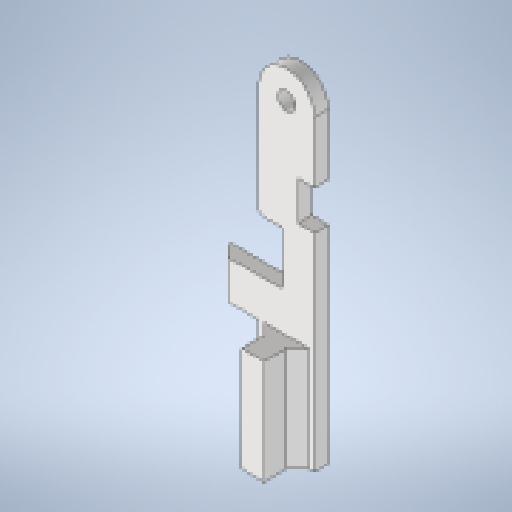
# Autodesk Inventor part: LatchLock
Saved by Autodesk Inventor 2025.1 (Build 291241000, 241)
## iProperties
Created: 2026-05-10
Part Number: LatchLock
Material: Generic
Document SubType Name: Modeling
Designer: User
Density: 1 g/cm^3
Appearance: Default
Author: User
Autodesk Inventor part; units mm, degrees
ref_plane "YZ Plane" through (0, 0, 0) normal (1, 0, 0) x (0, 1, 0)
ref_plane "XZ Plane" through (0, 0, 0) normal (0, 1, 0) x (-1, 0, 0)
ref_plane "XY Plane" through (0, 0, 0) normal (0, 0, 1) x (1, 0, 0)
sketch "Sketch1" plane through (0, 0, 0) normal (0, 0, 1) x (1, 0, 0)
  line L0 (8.404, 3) -> (8.404, -46.6888) projected
  line L1 (6.389, 0.2) -> (6.389, -55.1706) projected
  line L2 (7.404, -64.4706) -> (6.389, -64.4706) projected
  line L3 (6.389, -64.4706) -> (6.389, -78.3802) projected
  line L4 (-3.1786, -78.3802) -> (6.389, -78.3802) projected
  line L5 (-3.1786, -78.3802) -> (-3.1786, -81.1802) projected
  line L6 (8.404, -81.1802) -> (-3.1786, -81.1802) projected
  line L7 (8.404, -65.4706) -> (8.404, -81.1802) projected
  line L8 (8.604, -55.6706) -> (6.189, -55.6706)
  line L9 (6.189, -55.6706) -> (6.189, 0)
  line L10 (6.189, 0) -> (-3.3786, 0)
  line L11 (-3.3786, 0) -> (-3.3786, 3.2)
  line L12 (-3.3786, 3.2) -> (8.604, 3.2)
  line L13 (8.604, 3.2) -> (8.604, -55.6706)
  line L14 (8.604, -81.3802) -> (-3.3786, -81.3802)
  line L15 (-3.3786, -81.3802) -> (-3.3786, -78.1802)
  line L16 (-3.3786, -78.1802) -> (6.189, -78.1802)
  line L17 (6.189, -78.1802) -> (6.189, -64.2706)
  line L18 (6.189, -64.2706) -> (8.604, -64.2706)
  line L19 (8.604, -64.2706) -> (8.604, -81.3802)
  line L20 (13.604, -60.6706) -> (1.189, -60.6706)
  line L21 (1.189, -60.6706) -> (1.189, -5)
  line L22 (1.189, -5) -> (-8.3786, -5)
  line L23 (-8.3786, -5) -> (-8.3786, 8.2)
  line L24 (-8.3786, 8.2) -> (13.604, 8.2)
  line L25 (13.604, 8.2) -> (13.604, -60.6706)
  circle A0 centre (13.604, -26.2353) radius 5
  line L26 (18.604, -65.6706) -> (-3.811, -65.6706)
  line L27 (-3.811, -65.6706) -> (-3.811, -10)
  line L28 (-3.811, -10) -> (-13.3786, -10)
  line L29 (-13.3786, -10) -> (-13.3786, 13.2)
  line L30 (-13.3786, 13.2) -> (18.604, 13.2)
  line L31 (18.604, 13.2) -> (18.604, -65.6706)
  circle A1 centre (13.604, -26.2353) radius 1.6
  circle A2 centre (13.604, -26.2353) radius 30.3549
  circle A3 centre (13.604, -26.2353) radius 38.3626
  line L32 (8.604, -55.6706) -> (8.604, -56.1756)
  line L33 (6.189, -64.2706) -> (6.189, -63.8744)
  line L34 (6.189, -63.8744) -> (18.604, -63.8744)
  line L35 (6.189, -63.8744) -> (18.604, -63.8744) construction
  line L36 (8.604, -55.6706) -> (1.189, -55.6706)
  line L37 (1.189, -55.6706) -> (1.189, -63.8744)
  line L38 (1.189, -63.8744) -> (18.604, -63.8744)
  line L39 (1.189, -62.5334) -> (18.604, -62.5334)
  line L40 (1.189, -62.5334) -> (18.604, -62.5334) construction
  line L41 (6.389, -55.1706) -> (12.3969, -55.1706) projected
  line L42 (12.604, -54.9635) -> (12.3969, -55.1706) projected
  line L43 (12.604, -46.8959) -> (12.604, -54.9635) projected
  line L44 (12.3969, -46.6888) -> (12.604, -46.8959) projected
  line L45 (8.404, -46.6888) -> (12.3969, -46.6888) projected
  line L46 (-3.1786, 3) -> (8.404, 3) projected
  line L47 (-3.1786, 0.2) -> (-3.1786, 3) projected
  line L48 (-3.1786, 0.2) -> (6.389, 0.2) projected
  circle A4 centre (9.4965, -50.9297) radius 1.5 projected
  line L49 (7.404, -64.4706) -> (8.404, -65.4706) projected
  point P0 (0, 0)
  point P1 (8.604, -26.2353)
  point P2 (18.604, -26.2353)
  dimension "d0" = 0.2
  dimension "d1" = 0.2
  dimension "d2" = 5
  dimension "d3" = 5
  dimension "d4" = 3.2
  dimension "d5" = 0
  dimension "d6" = 0
  constraints: 66 end point, 6 point on line, 5 point on circle, 4 centre point, 3 coincident, 3 collinear, 2 horizontal, 1 midpoint, 1 parallel, 1 vertical, 15 other
  measures "d0" distance between parallel lines of L0 L13
  measures "d1" distance between parallel lines of L7 L19
  measures "d2" distance between parallel lines of L13 L25
  measures "d3" distance between parallel lines of L25 L31
  measures "d4" diameter of A1
  measures "d5" distance between parallel lines of L34 L35
  measures "d6" distance between parallel lines of L39 L40
extrude "Extrusion1" add sketch "Sketch1" along normal blind 2.5 contours L45 L44 L43 L42 L41 L13 A4 | L13 A0 L25 A2 L32 L41 L42 L43 L44 L45 | A0 L25 A1 | A4 L13 | A0 L25 A1 | A0 L31 A2 L25 | A2 L31 L39 L37 L20 L25 | L25 L20 L21 L36 A2 | L8 L32 A2 picked at (9.3865, -50.8083) picked at (16.7555, -47.8971)
sketch "Sketch2" plane through (1.189, -62.5334, 0) normal (0, -1, 0) x (1, 0, 0)
  line L0 (-0.8528, -0.0858) -> (2.6827, 3.4497) projected
  line L1 (-0.7114, -0.2272) -> (2.8241, 3.3083)
  line L2 (0, 2.5) -> (17.415, 2.5) projected
  line L3 (0, 0) -> (0, 2.5) projected
  point P0 (-1.189, 0)
  point P1 (0, 0.4842)
  point P2 (2.0158, 2.5)
  dimension "d9" = 0.2
  constraints: 2 end point, 1 parallel
  measures "d9" distance between parallel lines of L0 L1
extrude "Extrusion2" cut sketch "Sketch2" against normal through all
sketch "Sketch4" plane through (1.189, -62.5334, 0) normal (0, -1, 0) x (1, 0, 0)
  line L0 (2.0158, 2.5) -> (17.415, 2.5) projected
  line L1 (0, 0) -> (17.415, 0) projected
  line L2 (17.415, 0) -> (17.415, 2.5) projected
  line L3 (7.415, 0) -> (7.415, 2.5) projected
  point P0 (-1.189, 0)
ref_plane "Work Plane1" through (-8.1491, -81.1802, -17.0906) normal (0, -1, 0) x (0.7071068, 0, 0.7071068)
extrude "Extrusion3" add sketch "Sketch4" along normal up to surface (18.6468 mm away)
sketch "Sketch5" plane through (0, 0, 2.5) normal (0, 0, 1) x (1, 0, 0)
  line L0 (8.604, -26.2353) -> (8.604, -55.6706) projected
  circle A0 centre (13.604, -26.2353) radius 1.6 projected
  circle A1 centre (13.604, -26.2353) radius 29.857
  line L1 (8.604, -26.2353) -> (8.604, -55.6706) projected
  line L2 (8.604, -55.6706) -> (12.604, -55.6706)
  line L3 (8.604, -55.6706) -> (12.604, -55.6706) construction
  line L4 (12.604, -55.6706) -> (8.604, -55.6706)
  line L5 (8.604, -55.6706) -> (8.604, -51.6706)
  line L6 (8.604, -51.6706) -> (12.604, -51.6706)
  line L7 (12.604, -51.6706) -> (12.604, -55.6706)
  line L8 (12.604, -51.6706) -> (8.604, -51.6706)
  line L9 (8.604, -51.6706) -> (8.604, -47.6706)
  line L10 (8.604, -47.6706) -> (12.604, -47.6706)
  line L11 (12.604, -47.6706) -> (12.604, -51.6706)
  line L12 (12.604, -47.6706) -> (8.604, -47.6706)
  line L13 (8.604, -47.6706) -> (8.604, -46.6706)
  line L14 (8.604, -46.6706) -> (12.604, -46.6706)
  line L15 (12.604, -46.6706) -> (12.604, -47.6706)
  circle A2 centre (13.604, -26.2353) radius 20.4598
  circle A3 centre (13.604, -26.2353) radius 19.9598
  line L16 (12.604, -55.6706) -> (13.104, -55.6706)
  line L17 (13.104, -55.6706) -> (13.104, -46.1888)
  line L18 (13.104, -46.1888) -> (8.604, -46.1888)
  point P0 (0, 0)
  dimension "d22" = 0.5
  dimension "d14" = 4
  dimension "d15" = 0
  dimension "d16" = 4
  dimension "d17" = 4
  dimension "d18" = 4
  dimension "d19" = 4
  dimension "d20" = 4
  dimension "d21" = 1
  dimension "d23" = 0.5
  dimension "d24" = 90
  dimension "d25" = 90
  constraints: 34 end point, 6 parallel, 4 horizontal, 4 perpendicular, 2 coincident, 2 point on line, 1 collinear, 9 other
  measures "d14" distance of L0.end L2.end
  measures "d15" distance between parallel lines of L2 L3
  measures "d16" distance of L5.end L6.end
  measures "d17" distance of L4.end L5.end
  measures "d18" distance of L9.end L10.end
  measures "d19" distance of L8.end L9.end
  measures "d20" distance of L13.end L14.end
  measures "d21" distance of L12.end L13.end
  measures "d23" distance of L3.end L16.end
  measures "d24" angle of L17 L16
  measures "d25" angle of L18 L17
extrude "Extrusion4" cut sketch "Sketch5" against normal blind 10 contours L18 A2 L14 L0 | L14 L15 L10 L0 | L18 L17 A2 | L10 L11 L6 L0 | A2 L17 L16 L7 L11 L15 | L6 L7 L2 L0
chamfer "Chamfer1" distance 0.5 angle 45 3 edges at (8.604, -46.1888, 1.25) (13.104, -46.1888, 1.25) (13.104, -55.6706, 1.25)
sketch "Sketch6" plane through (0, 0, 2.5) normal (0, 0, 1) x (1, 0, 0)
  line L0 (18.604, -26.2353) -> (18.604, -81.1802) projected
  line L1 (8.604, -62.5334) -> (8.604, -81.1802) projected
  line L2 (15.604, -26.2353) -> (15.604, -81.1802)
  line L3 (11.604, -62.5334) -> (11.604, -81.1802)
  line L4 (11.604, -62.5334) -> (15.604, -62.5334)
  line L5 (15.604, -62.5334) -> (15.604, -81.1802)
  line L6 (15.604, -81.1802) -> (11.604, -81.1802)
  line L7 (11.604, -81.1802) -> (11.604, -62.5334)
  point P0 (0, 0)
  dimension "d31" = 3
  dimension "d32" = 3
  constraints: 12 end point, 4 parallel, 1 horizontal, 1 perpendicular
  measures "d31" distance between parallel lines of L0 L2
  measures "d32" distance between parallel lines of L1 L3
extrude "Extrusion5" add sketch "Sketch6" along normal blind 6
chamfer "Chamfer2" distance 2 angle 45 2 edges at (11.604, -71.8568, 2.5) (15.604, -71.8568, 2.5)
sketch "Sketch7" plane through (0, 0, 2.5) normal (0, 0, 1) x (1, 0, 0)
  line L0 (18.604, -26.2353) -> (18.604, -81.1802) projected
  line L1 (9.104, -46.1888) -> (12.604, -46.1888) projected
  line L2 (9.104, -44.1888) -> (12.604, -44.1888)
  line L3 (18.604, -44.1888) -> (15.604, -44.1888)
  line L4 (15.604, -44.1888) -> (15.604, -37.1888)
  line L5 (15.604, -37.1888) -> (18.604, -37.1888)
  line L6 (18.604, -37.1888) -> (18.604, -44.1888)
  point P0 (0, 0)
  dimension "d38" = 2
  dimension "d39" = 3
  dimension "d40" = 7
  constraints: 10 end point, 3 parallel, 1 horizontal, 1 perpendicular, 1 point on line
  measures "d38" distance between parallel lines of L1 L2
  measures "d39" distance of L4.end L5.end
  measures "d40" distance of L3.end L4.end
extrude "Extrusion6" cut sketch "Sketch7" against normal blind 6
sketch "Sketch9" plane through (1.189, -62.5334, 0) normal (0, -1, 0) x (1, 0, 0)
  line L0 (2.0158, 2.5) -> (7.415, 2.5) projected
  line L1 (2.0158, 2.5) -> (0, 0.4842) projected
  line L2 (7.415, 0) -> (7.415, 2.5) projected
  line L3 (7.415, 2.5) -> (7.415, 5.5)
  line L4 (7.415, 2.5) -> (10.415, 2.5) construction
  line L5 (0, 0.4842) -> (5.0158, 5.5)
  line L6 (17.415, 2.5) -> (17.415, 0) projected
  line L7 (5.0158, 5.5) -> (17.415, 5.5)
  line L8 (5.0158, 5.5) -> (17.415, 5.5) construction
  line L9 (17.415, 5.5) -> (17.415, 2.5)
  line L10 (17.415, 2.5) -> (7.415, 2.5)
  point P0 (-1.189, 0)
  dimension "d43" = 3
  dimension "d44" = 90
  dimension "d45" = 0
  constraints: 14 end point, 2 equal length, 2 horizontal, 2 perpendicular, 1 vertical
  measures "d43" distance of L0.end L3.end
  measures "d44" angle of L4 L3
  measures "d45" distance between parallel lines of L7 L8
extrude "Extrusion7" add sketch "Sketch9" against normal blind 3
chamfer "Chamfer3" distance 2 angle 45 1 edges at (18.604, -59.5334, 4)
chamfer "Chamfer4" distance 3 angle 45 1 edges at (13.604, -62.5334, 5.5)
body "Solid1"
